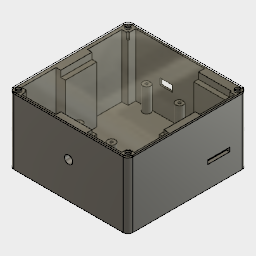
Pixel v11 (Autodesk Fusion 360 design; units mm, degrees)
Autodesk Fusion 360 part; units mm, degrees
note: some values were not read from the file. Set by a fixed rule: which sketch regions a step uses.
sketch "Sketch1" plane through (0, 0, 0) normal (0, 1, 0) x (1, 0, 0) in component "Box"
  line L0 (33, 33) -> (-33, 33)
  line L1 (-33, 33) -> (-33, -33)
  line L2 (-33, -33) -> (33, -33)
  line L3 (33, -33) -> (33, 33)
  line L4 (33, 33) -> (-33, -33) construction
  line L5 (-33, 33) -> (33, -33) construction
  line L6 (38, 38) -> (-38, 38)
  line L7 (-38, 38) -> (-38, -38)
  line L8 (-38, -38) -> (38, -38)
  line L9 (38, -38) -> (38, 38)
  line L10 (38, 38) -> (-38, -38) construction
  line L11 (-38, 38) -> (38, -38) construction
  dimension "d1" = 66
  dimension "d2" = 66
  dimension "d3" = 76
  dimension "d4" = 76
  measures "d1" distance of L1.end L2.end
  measures "d2" distance of L0.end L1.end
  measures "d3" distance of L6.end L7.end
  measures "d4" distance of L7 L9
extrude "Extrude1" add sketch "Sketch1" along normal blind 2 contours L0 L1 L2 L3 | L6 L7 L8 L9 makes body 1 in component "Box"
sketch "Sketch2" plane through (0, 2, 0) normal (0, 1, 0) x (-1, 0, 0) in component "Box"
  line L0 (-38, 38) -> (-38, -38)
  line L1 (-38, -38) -> (38, -38)
  line L2 (38, -38) -> (38, 38)
  line L3 (38, 38) -> (-38, 38)
  line L4 (36, -36) -> (36, 36)
  line L5 (36, 36) -> (-36, 36)
  line L6 (-36, 36) -> (-36, -36)
  line L7 (-36, -36) -> (36, -36)
  dimension "d7" = 2
extrude "Extrude2" add sketch "Sketch2" along normal blind 40 bodies 1 in component "Box"
sketch "Sketch3" plane through (0, 2, 0) normal (0, 1, 0) x (-1, 0, 0) in component "Box"
  line L0 (36, -36) -> (36, 36)
  line L1 (36, 36) -> (-36, 36)
  line L2 (-36, 36) -> (-36, -36)
  line L3 (-36, -36) -> (36, -36)
  line L4 (-36, -36) -> (-32, -36)
  line L5 (-32, -36) -> (-32, -32)
  line L6 (-32, -32) -> (-36, -32)
  line L7 (-36, -32) -> (-36, -36)
  dimension "d10" = 4
  dimension "d11" = 4
  measures "d10" distance of L2.end L4.end
  measures "d11" distance of L4 L6
extrude "Extrude3" add sketch "Sketch3" along normal blind 40 contours L2 L3 L4 L5 L6 L7 bodies 1 in component "Box"
mirror "Mirror1" about plane through (0, 0, 0) normal (0, 0, 1) of "Extrude3" in component "Box"
mirror "Mirror2" about plane through (0, 0, 0) normal (1, 0, 0) of "Extrude3", "Mirror1" in component "Box"
sketch "Sketch4" plane through (0, 42, 0) normal (0, 1, 0) x (-1, 0, 0) in component "Box"
  line L0 (32, -36) -> (-32, -36)
  line L1 (-32, -36) -> (-32, -32)
  line L2 (-32, -32) -> (-36, -32)
  line L3 (-36, -32) -> (-36, 32)
  line L4 (-36, 32) -> (-32, 32)
  line L5 (-32, 32) -> (-32, 36)
  line L6 (-32, 36) -> (32, 36)
  line L7 (32, 36) -> (32, 32)
  line L8 (32, 32) -> (36, 32)
  line L9 (36, 32) -> (36, -32)
  line L10 (36, -32) -> (32, -32)
  line L11 (32, -32) -> (32, -36)
  line L12 (38, 38) -> (-38, 38)
  line L13 (-38, 38) -> (-38, -38)
  line L14 (-38, -38) -> (38, -38)
  line L15 (38, -38) -> (38, 38)
  circle A0 centre (-35, -35) radius 1.5
  dimension "d16" = 3
  dimension "d17" = 3
  dimension "d18" = 3
  measures "d16" diameter of A0
  measures "d17" distance of L2 A0.centre
  measures "d18" distance of L1 A0.centre
extrude "Extrude4" cut sketch "Sketch4" against normal blind 20 contours A0 bodies 1 in component "Box"
mirror "Mirror3" about plane through (0, 0, 0) normal (0, 0, 1) of "Extrude4" in component "Box"
mirror "Mirror4" about plane through (0, 0, 0) normal (1, 0, 0) of "Extrude4", "Mirror3" in component "Box"
sketch "Sketch5" plane through (0, 42, 0) normal (0, 1, 0) x (-1, 0, 0) in component "Box"
  circle A0 centre (35, 35) radius 1.5
  circle A1 centre (35, -35) radius 1.5
  circle A2 centre (-35, 35) radius 1.5
  circle A3 centre (-35, -35) radius 1.5
  line L0 (32, -36) -> (-32, -36)
  line L1 (-32, -36) -> (-32, -32)
  line L2 (-32, -32) -> (-36, -32)
  line L3 (-36, -32) -> (-36, 32)
  line L4 (-36, 32) -> (-32, 32)
  line L5 (-32, 32) -> (-32, 36)
  line L6 (-32, 36) -> (32, 36)
  line L7 (32, 36) -> (32, 32)
  line L8 (32, 32) -> (36, 32)
  line L9 (36, 32) -> (36, -32)
  line L10 (36, -32) -> (32, -32)
  line L11 (32, -32) -> (32, -36)
  line L12 (38, 38) -> (-38, 38)
  line L13 (-38, 38) -> (-38, -38)
  line L14 (-38, -38) -> (38, -38)
  line L15 (38, -38) -> (38, 38)
  line L16 (30, -30) -> (30, 30)
  line L17 (30, 30) -> (-30, 30)
  line L18 (-30, 30) -> (-30, -30)
  line L19 (-30, -30) -> (30, -30)
  line L20 (-30, -10) -> (-38, -10)
  line L21 (-38, -10) -> (-38, 10)
  line L22 (-38, 10) -> (-30, 10)
  line L23 (-30, 10) -> (-30, -10)
  line L24 (-10, 38) -> (10, 38)
  line L25 (10, 38) -> (10, 30)
  line L26 (10, 30) -> (-10, 30)
  line L27 (-10, 30) -> (-10, 38)
  dimension "d23" = 8
  dimension "d24" = 28
  dimension "d25" = 20
  dimension "d29" = 20
  dimension "d30" = 28
  dimension "d35" = 8
  measures "d24" distance of L14 L20
  measures "d25" distance of L20 L22
  measures "d29" distance of L25 L27
  measures "d30" distance of L13 L27
  measures "d35" distance of L17 L24
extrude "Extrude6" add sketch "Sketch5" against normal blind 40 contours L3 L18 L20 L22 L23 | L6 L17 L25 L26 L27 bodies 1 in component "Box"
mirror "Mirror6" about plane through (0, 0, 0) normal (1, 0, 0) of "Extrude6" in component "Box"
sketch "Sketch8" plane through (0, 42, 0) normal (0, 1, 0) x (-1, 0, 0) in component "Box"
  line L0 (-36, 10) -> (-36, 32)
  line L1 (-36, 32) -> (-32, 32)
  line L2 (-32, 32) -> (-32, 36)
  line L3 (-32, 36) -> (-10, 36)
  line L4 (-10, 36) -> (-10, 30)
  line L5 (-10, 30) -> (10, 30)
  line L6 (10, 30) -> (10, 36)
  line L7 (10, 36) -> (32, 36)
  line L8 (32, 36) -> (32, 32)
  line L9 (32, 32) -> (36, 32)
  line L10 (36, 32) -> (36, 10)
  line L11 (36, 10) -> (30, 10)
  line L12 (30, 10) -> (30, -10)
  line L13 (30, -10) -> (36, -10)
  line L14 (36, -10) -> (36, -32)
  line L15 (36, -32) -> (32, -32)
  line L16 (32, -32) -> (32, -36)
  line L17 (32, -36) -> (-32, -36)
  line L18 (-32, -36) -> (-32, -32)
  line L19 (-32, -32) -> (-36, -32)
  line L20 (-36, -32) -> (-36, -10)
  line L21 (-36, -10) -> (-30, -10)
  line L22 (-30, -10) -> (-30, 10)
  line L23 (-30, 10) -> (-36, 10)
  line L24 (38, 38) -> (-38, 38)
  line L25 (-38, 38) -> (-38, -38)
  line L26 (-38, -38) -> (38, -38)
  line L27 (38, -38) -> (38, 38)
  circle A0 centre (-35, -35) radius 1.5
  circle A1 centre (-35, 35) radius 1.5
  circle A2 centre (35, -35) radius 1.5
  circle A3 centre (35, 35) radius 1.5
  line L28 (33, -33) -> (33, 33)
  line L29 (33, 33) -> (-33, 33)
  line L30 (-33, 33) -> (-33, -33)
  line L31 (-33, -33) -> (33, -33)
  dimension "d37" = 5
extrude "Extrude9" cut sketch "Sketch8" against normal blind 4 contours L1 L2 L4 L5 L6 L8 L9 L11 L12 L13 L15 L16 L18 L19 L21 L22 L23 L28 L29 L30 L31 | L21 L22 L23 L30 | L1 L2 L29 L30 | L18 L19 L30 L31 | L4 L5 L6 L29 | L15 L16 L28 L31 | L8 L9 L28 L29 | L11 L12 L13 L28 bodies 1 in component "Box"
sketch "Sketch9" plane through (0, 2, 0) normal (0, 1, 0) x (-1, 0, 0) in component "Box"
  line L0 (32, 32) -> (32, 36)
  line L1 (32, 36) -> (10, 36)
  line L2 (-32, 36) -> (-32, 32)
  line L3 (-32, 32) -> (-36, 32)
  line L4 (-36, 32) -> (-36, 10)
  line L5 (-36, -32) -> (-32, -32)
  line L6 (-32, -32) -> (-32, -36)
  line L7 (-32, -36) -> (32, -36)
  line L8 (32, -36) -> (32, -32)
  line L9 (32, -32) -> (36, -32)
  line L10 (36, 10) -> (36, 32)
  line L11 (36, 32) -> (32, 32)
  line L12 (-32, -36) -> (-12, -36)
  line L13 (-12, -36) -> (-12, -30)
  line L14 (-12, -30) -> (-32, -30)
  line L15 (-32, -30) -> (-32, -36)
  line L16 (30, 10) -> (36, 10)
  line L17 (10, 36) -> (10, 30)
  line L18 (10, 30) -> (-10, 30)
  line L19 (-10, 30) -> (-10, 36)
  line L20 (-10, 36) -> (-32, 36)
  line L21 (-36, 10) -> (-30, 10)
  line L22 (-30, 10) -> (-30, -10)
  line L23 (-30, -10) -> (-36, -10)
  line L24 (-36, -10) -> (-36, -32)
  line L25 (36, -32) -> (36, -10)
  line L26 (36, -10) -> (30, -10)
  line L27 (30, -10) -> (30, 10)
  dimension "d44" = 20
  measures "d44" distance of L6.end L12.end
extrude "Extrude10" add sketch "Sketch9" along normal blind 36 contours L6 L7 L12 L13 L14 L15 bodies 1 in component "Box"
sketch "Sketch10" plane through (0, 38, 0) normal (0, 1, 0) x (-1, 0, 0) in component "Box"
  line L0 (-32, -32) -> (-33, -32)
  line L1 (-33, -32) -> (-33, -33)
  line L2 (-33, -33) -> (-32, -33)
  line L3 (-32, -33) -> (-32, -36)
  line L4 (-32, -36) -> (-12, -36)
  line L5 (-12, -36) -> (-12, -30)
  line L6 (-12, -30) -> (-32, -30)
  line L7 (-32, -30) -> (-32, -32)
  line L8 (-32, -36) -> (-12, -36)
  line L9 (-12, -36) -> (-12, -33)
  line L10 (-12, -33) -> (-32, -33)
  line L11 (-32, -33) -> (-32, -36)
extrude "Extrude11" add sketch "Sketch10" along normal blind 4 contours L3 L4 L5 L8 L9 L10 L11 bodies 1 in component "Box"
sketch "Sketch13" plane through (0, 42, 0) normal (0, 1, 0) x (-1, 0, 0) in component "Box"
  circle A0 centre (35, 35) radius 1.5
  circle A1 centre (35, -35) radius 1.5
  circle A2 centre (-35, 35) radius 1.5
  circle A3 centre (-35, -35) radius 1.5
  line L0 (38, 38) -> (-38, 38)
  line L1 (-38, 38) -> (-38, -38)
  line L2 (-38, -38) -> (38, -38)
  line L3 (38, -38) -> (38, 38)
  line L4 (33, -32) -> (33, -33)
  line L5 (33, -33) -> (32, -33)
  line L6 (32, -33) -> (32, -36)
  line L7 (32, -36) -> (-12, -36)
  line L8 (-12, -36) -> (-12, -33)
  line L9 (-12, -33) -> (-33, -33)
  line L10 (-33, -33) -> (-33, -32)
  line L11 (-33, -32) -> (-36, -32)
  line L12 (-36, -32) -> (-36, -10)
  line L13 (-36, -10) -> (-33, -10)
  line L14 (-33, -10) -> (-33, 10)
  line L15 (-33, 10) -> (-36, 10)
  line L16 (-36, 10) -> (-36, 32)
  line L17 (-36, 32) -> (-33, 32)
  line L18 (-33, 32) -> (-33, 33)
  line L19 (-33, 33) -> (-32, 33)
  line L20 (-32, 33) -> (-32, 36)
  line L21 (-32, 36) -> (-10, 36)
  line L22 (-10, 36) -> (-10, 33)
  line L23 (-10, 33) -> (10, 33)
  line L24 (10, 33) -> (10, 36)
  line L25 (10, 36) -> (32, 36)
  line L26 (32, 36) -> (32, 33)
  line L27 (32, 33) -> (33, 33)
  line L28 (33, 33) -> (33, 32)
  line L29 (33, 32) -> (36, 32)
  line L30 (36, 32) -> (36, 10)
  line L31 (36, 10) -> (33, 10)
  line L32 (33, 10) -> (33, -10)
  line L33 (33, -10) -> (36, -10)
  line L34 (36, -10) -> (36, -32)
  line L35 (36, -32) -> (33, -32)
  line L36 (32, -36) -> (-12, -36)
  line L37 (-12, -36) -> (-12, -37)
  line L38 (-12, -37) -> (32, -37)
  line L39 (32, -37) -> (32, -36)
  dimension "d55" = 1
  measures "d55" distance of L6.end L38.end
extrude "Extrude13" cut sketch "Sketch13" against normal blind 40 contours L7 L36 L37 L38 L39 bodies 1 in component "Box"
sketch "Sketch14" plane through (0, 2, 0) normal (0, 1, 0) x (-1, 0, 0) in component "Box"
  line L0 (-12, -30) -> (-12, -37)
  line L1 (-12, -37) -> (32, -37)
  line L2 (32, -37) -> (32, -32)
  line L3 (32, -32) -> (36, -32)
  line L4 (36, -32) -> (36, -10)
  line L5 (36, 32) -> (32, 32)
  line L6 (32, 32) -> (32, 36)
  line L7 (32, 36) -> (10, 36)
  line L8 (-32, 36) -> (-32, 32)
  line L9 (-32, 32) -> (-36, 32)
  line L10 (-36, 32) -> (-36, 10)
  line L11 (-36, -32) -> (-32, -32)
  line L12 (-32, -32) -> (-32, -30)
  line L13 (-32, -30) -> (-12, -30)
  line L14 (23, -35) -> (2, -35)
  line L15 (2, -35) -> (2, 8.5)
  line L16 (2, 8.5) -> (23, 8.5)
  line L17 (23, 8.5) -> (23, -35)
  circle A0 centre (23, -35) radius 0.8
  circle A1 centre (23, 8.5) radius 0.8
  circle A2 centre (2, 8.5) radius 0.8
  circle A3 centre (2, -35) radius 0.8
  circle A4 centre (2, 8.5) radius 2.5
  circle A5 centre (23, 8.5) radius 2.5
  circle A6 centre (23, -35) radius 2.5
  circle A7 centre (2, -35) radius 2.5
  line L18 (36, -10) -> (30, -10)
  line L19 (30, -10) -> (30, 10)
  line L20 (30, 10) -> (36, 10)
  line L21 (36, 10) -> (36, 32)
  line L22 (10, 36) -> (10, 30)
  line L23 (10, 30) -> (-10, 30)
  line L24 (-10, 30) -> (-10, 36)
  line L25 (-10, 36) -> (-32, 36)
  line L26 (-36, 10) -> (-30, 10)
  line L27 (-30, 10) -> (-30, -10)
  line L28 (-30, -10) -> (-36, -10)
  line L29 (-36, -10) -> (-36, -32)
  dimension "d58" = 21
  dimension "d59" = 43.5
  dimension "d60" = 2
  dimension "d61" = 13
  dimension "d62" = 1.6
  dimension "d63" = 1.6
  dimension "d64" = 1.6
  dimension "d65" = 1.6
  dimension "d66" = 5
  dimension "d67" = 5
  dimension "d68" = 5
  dimension "d69" = 5
  measures "d58" distance of L14.start L14.end
  measures "d59" distance of L14.start L16.end
  measures "d60" distance of L1 L14
  measures "d61" distance of L4 L17
  measures "d62" diameter of A0
  measures "d63" diameter of A1
  measures "d64" diameter of A2
  measures "d65" diameter of A3
  measures "d66" diameter of A4
  measures "d67" diameter of A5
  measures "d68" diameter of A6
  measures "d69" diameter of A7
extrude "Extrude14" add sketch "Sketch14" along normal blind 15 contours L1 L14 L15 A3 A7 | L1 A7 | L14 L15 A3 A7 | L1 L14 L17 A0 A6 | L1 A6 | L15 L16 A2 A4 | L15 L16 A2 A4 | L14 L17 A0 A6 | L16 L17 A1 A5 | L16 L17 A1 A5 bodies 1 in component "Box"
sketch "Sketch15" plane through (0, 0, -37) normal (0, 0, 1) x (1, 0, 0) in component "Box"
  line L0 (-3.5, 2) -> (-3.5, 17)
  line L1 (-3.5, 17) -> (-0.5, 17)
  line L2 (-0.5, 17) -> (-0.5, 2)
  line L3 (-0.5, 2) -> (12, 2)
  line L4 (12, 2) -> (12, 42)
  line L5 (12, 42) -> (-32, 42)
  line L6 (-32, 42) -> (-32, 2)
  line L7 (-32, 2) -> (-24.5, 2)
  line L8 (-24.5, 2) -> (-24.5, 17)
  line L9 (-24.5, 17) -> (-21.5, 17)
  line L10 (-21.5, 17) -> (-21.5, 2)
  line L11 (-21.5, 2) -> (-3.5, 2)
  line L12 (-2, 17) -> (-23, 17) construction
  line L13 (-16.5, 18.5) -> (-8.5, 18.5)
  line L14 (-8.5, 18.5) -> (-8.5, 22.5)
  line L15 (-8.5, 22.5) -> (-16.5, 22.5)
  line L16 (-16.5, 22.5) -> (-16.5, 18.5)
  dimension "d72" = 8
  dimension "d73" = 4
  dimension "d74" = 1.5
  dimension "d75" = 15.5
  measures "d72" distance of L13.start L13.end
  measures "d73" distance of L13.start L15.end
  measures "d74" distance of L12 L13
  measures "d75" distance of L6 L16
extrude "Extrude15" cut sketch "Sketch15" against normal up to surface (1 mm away) contours L13 L14 L15 L16 bodies 1 in component "Box"
fillet "Fillet1" radius 3 4 edges at (38, 21, 38) (-38, 21, 38) (38, 21, -38) (-38, 21, -38) on bodies 1 in component "Box"
sketch "Sketch16" plane through (0, 2, 0) normal (0, 1, 0) x (-1, 0, 0) in component "Box"
  circle A0 centre (2, 8.5) radius 2.5
  arc A1 (3.5, -37) -> (0.5, -37) centre (2, -35) ccw
  line L0 (3.5, -37) -> (21.5, -37)
  arc A2 (24.5, -37) -> (21.5, -37) centre (23, -35) ccw
  line L1 (24.5, -37) -> (32, -37)
  line L2 (32, -37) -> (32, -32)
  line L3 (32, -32) -> (36, -32)
  line L4 (36, -32) -> (36, -10)
  line L5 (36, 32) -> (32, 32)
  line L6 (32, 32) -> (32, 36)
  line L7 (32, 36) -> (10, 36)
  line L8 (-32, 36) -> (-32, 32)
  line L9 (-32, 32) -> (-36, 32)
  line L10 (-36, 32) -> (-36, 10)
  line L11 (-36, -32) -> (-32, -32)
  line L12 (-32, -32) -> (-32, -30)
  line L13 (-32, -30) -> (-12, -30)
  line L14 (-12, -30) -> (-12, -37)
  line L15 (-12, -37) -> (0.5, -37)
  circle A3 centre (23, 8.5) radius 2.5
  line L16 (-20.5, -30) -> (-36, -30)
  line L17 (-36, -30) -> (-36, -10)
  line L18 (-36, -10) -> (-20.5, -10)
  line L19 (-20.5, -10) -> (-20.5, -30)
  line L20 (36, -10) -> (30, -10)
  line L21 (30, -10) -> (30, 10)
  line L22 (30, 10) -> (36, 10)
  line L23 (36, 10) -> (36, 32)
  line L24 (10, 36) -> (10, 30)
  line L25 (10, 30) -> (-10, 30)
  line L26 (-10, 30) -> (-10, 36)
  line L27 (-10, 36) -> (-32, 36)
  line L28 (-36, 10) -> (-30, 10)
  line L29 (-30, 10) -> (-30, -10)
  line L30 (-30, -10) -> (-36, -10)
  line L31 (-36, -10) -> (-36, -32)
  dimension "d79" = 15.5
  dimension "d80" = 20
  dimension "d82" = 56.5
  dimension "d88" = 2
  measures "d79" distance of L16.start L16.end
  measures "d80" distance of L16 L18
  measures "d82" distance of L4 L19
  measures "d88" distance of L11 L16
extrude "Extrude17" add sketch "Sketch16" along normal blind 10 contours L13 L16 L17 L18 L19 L30 L31 | L11 L12 L16 L31 bodies 1 in component "Box"
sketch "Sketch18" plane through (0, 12, 0) normal (0, 1, 0) x (-1, 0, 0) in component "Box"
  line L0 (-20.5, -10) -> (-30, -10)
  line L1 (-30, -10) -> (-36, -10)
  line L2 (-36, -10) -> (-36, -32)
  line L3 (-36, -32) -> (-32, -32)
  line L4 (-32, -32) -> (-32, -30)
  line L5 (-32, -30) -> (-20.5, -30)
  line L6 (-20.5, -30) -> (-20.5, -10)
  line L7 (-32, -30) -> (-36, -30)
extrude "Extrude18" add sketch "Sketch18" along normal blind 26 contours L2 L3 L4 L7 bodies 1 in component "Box"
sketch "Sketch19" plane through (0, 12, 0) normal (0, 1, 0) x (-1, 0, 0) in component "Box"
  line L0 (-36, -30) -> (-20.5, -30)
  line L1 (-20.5, -30) -> (-20.5, -10)
  line L2 (-20.5, -10) -> (-30, -10)
  line L3 (-30, -10) -> (-36, -10)
  line L4 (-36, -10) -> (-36, -30)
  circle A0 centre (-22, -27.25) radius 0.8
  line L5 (-22, -27.25) -> (-22, -12.75)
  circle A1 centre (-22, -12.75) radius 0.8
  dimension "d93" = 1.6
  dimension "d94" = 14.5
  dimension "d95" = 1.6
  dimension "d96" = 14
  dimension "d97" = 2.75
  measures "d93" diameter of A0
  measures "d94" distance of A0.centre L5.end
  measures "d95" diameter of A1
  measures "d96" distance of L4 L5
  measures "d97" distance of L2 L5.end
extrude "Extrude19" cut sketch "Sketch19" against normal blind 6 contours A0 | A1 bodies 1 in component "Box"
sketch "Sketch20" plane through (36, 0, 0) normal (-1, 0, 0) x (0, 0, 1) in component "Box"
  line L0 (-32, 38) -> (-30, 38)
  line L1 (-30, 38) -> (-30, 12)
  line L2 (-30, 12) -> (-10, 12)
  line L3 (-10, 12) -> (-10, 42)
  line L4 (-10, 42) -> (-32, 42)
  line L5 (-32, 42) -> (-32, 38)
  line L6 (-27, 13.8) -> (-13, 13.8)
  line L7 (-13, 13.8) -> (-13, 16.3)
  line L8 (-13, 16.3) -> (-27, 16.3)
  line L9 (-27, 16.3) -> (-27, 13.8)
  dimension "d100" = 14
  dimension "d101" = 2.5
  dimension "d102" = 3
  dimension "d103" = 1.8
  measures "d100" distance of L6.start L6.end
  measures "d101" distance of L6.start L8.end
  measures "d102" distance of L3 L7
  measures "d103" distance of L2 L6
extrude "Extrude20" cut sketch "Sketch20" against normal up to surface (2 mm away) contours L6 L7 L8 L9 bodies 1 in component "Box"
sketch "Sketch21" plane through (0, 0, 30) normal (0, 0, -1) x (-1, 0, 0) in component "Box"
  line L0 (10, 38) -> (-10, 38)
  line L1 (-10, 38) -> (-10, 2)
  line L2 (-10, 2) -> (10, 2)
  line L3 (10, 2) -> (10, 38)
  circle A0 centre (0, 23) radius 2.6
  dimension "d106" = 5.2
  dimension "d107" = 10
  dimension "d108" = 15
  measures "d106" diameter of A0
  measures "d107" distance of L3 A0.centre
  measures "d108" distance of L0 A0.centre
extrude "Extrude21" cut sketch "Sketch21" against normal up to surface (8 mm away) contours A0 bodies 1 in component "Box"
sketch "Sketch8 (2)" plane through (0, 42, 0) normal (0, 1, 0) x (-1, 0, 0) in component "Lid"
  line L0 (32, -33) -> (32, -37)
  line L1 (32, -37) -> (-12, -37)
  line L2 (-12, -37) -> (-12, -33)
  line L3 (-12, -33) -> (-33, -33)
  line L4 (-33, -33) -> (-33, -32)
  line L5 (-33, -32) -> (-36, -32)
  line L6 (-36, -32) -> (-36, -10)
  line L7 (-36, -10) -> (-33, -10)
  line L8 (-33, -10) -> (-33, 10)
  line L9 (-33, 10) -> (-36, 10)
  line L10 (-36, 10) -> (-36, 32)
  line L11 (-36, 32) -> (-33, 32)
  line L12 (-33, 32) -> (-33, 33)
  line L13 (-33, 33) -> (-32, 33)
  line L14 (-32, 33) -> (-32, 36)
  line L15 (-32, 36) -> (-10, 36)
  line L16 (-10, 36) -> (-10, 33)
  line L17 (-10, 33) -> (10, 33)
  line L18 (10, 33) -> (10, 36)
  line L19 (10, 36) -> (32, 36)
  line L20 (32, 36) -> (32, 33)
  line L21 (32, 33) -> (33, 33)
  line L22 (33, 33) -> (33, 32)
  line L23 (33, 32) -> (36, 32)
  line L24 (36, 32) -> (36, 10)
  line L25 (36, 10) -> (33, 10)
  line L26 (33, 10) -> (33, -10)
  line L27 (33, -10) -> (36, -10)
  line L28 (36, -10) -> (36, -32)
  line L29 (36, -32) -> (33, -32)
  line L30 (33, -32) -> (33, -33)
  line L31 (33, -33) -> (32, -33)
  arc A0 (35, -38) -> (38, -35) centre (35, -35) ccw
  line L32 (38, -35) -> (38, 35)
  arc A1 (38, 35) -> (35, 38) centre (35, 35) ccw
  line L33 (35, 38) -> (-35, 38)
  arc A2 (-35, 38) -> (-38, 35) centre (-35, 35) ccw
  line L34 (-38, 35) -> (-38, -35)
  arc A3 (-38, -35) -> (-35, -38) centre (-35, -35) ccw
  line L35 (-35, -38) -> (35, -38)
  circle A4 centre (-35, -35) radius 1.5
  circle A5 centre (-35, 35) radius 1.5
  circle A6 centre (35, -35) radius 1.5
  circle A7 centre (35, 35) radius 1.5
  line L36 (-35, -38) -> (35, -38)
  arc A8 (-38, -35) -> (-35, -38) centre (-35, -35) ccw
  line L37 (-38, 35) -> (-38, -35)
  circle A9 centre (-35, -35) radius 1.5
  circle A10 centre (35, -35) radius 1.5
  arc A11 (35, -38) -> (38, -35) centre (35, -35) ccw
  line L38 (38, -35) -> (38, 35)
  line L39 (35, 38) -> (-35, 38)
  arc A12 (38, 35) -> (35, 38) centre (35, 35) ccw
  circle A13 centre (35, 35) radius 1.5
  circle A14 centre (-35, 35) radius 1.5
extrude "Extrude7" add sketch "Sketch8 (2)" along normal blind 1 separate body contours L0 L1 L2 L3 L4 L5 L6 L7 L8 L9 L10 L11 L12 L13 L14 L15 L16 L17 L18 L19 L20 L21 L22 L23 L24 L25 L26 L27 L28 L29 L30 L31 | A0 L32 A1 L33 A2 L34 A3 L35 L36 A8 L37 A11 L38 L39 A12 makes body 2 in component "Lid"
component "Box" placed x (1, 0, 0) y (0, 1, 0) z (0, 0, 1) at (0, 0, 0)
component "Lid" placed x (1, 0, 0) y (0, 1, 0) z (0, 0, 1) at (0, 0, 0)
named bodies: "box", "lid"
